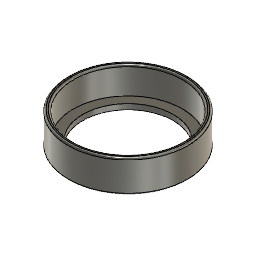
16) PLA Flexure Housing Ring 0.2mm Offset S2 (Autodesk Fusion 360 design; units mm, degrees)
Autodesk Fusion 360 part; units mm, degrees
sketch "Sketch1" plane through (0, 0, 0) normal (0, 0, 1) x (1, 0, 0)
  circle A0 centre (0, 0) radius 25
  circle A1 centre (0, 0) radius 30
  circle A2 centre (0, 0) radius 33
  dimension "d1" = 50
  dimension "d2" = 60
  dimension "d3" = 66
  constraint coincident A0.centre A1.centre
  constraint concentric A0 A1
  measures "d1" diameter of A0
  measures "d2" diameter of A1
  measures "d3" diameter of A2
extrude "Extrude1" add sketch "Sketch1" along normal blind 3 contours A1 | A2
sketch "Sketch2" plane through (0, 0, 3) normal (0, 0, 1) x (-1, 0, 0)
  circle A0 centre (0, 0) radius 25
  circle A1 centre (0, 0) radius 33
  circle A2 centre (0, 0) radius 30
  circle A3 centre (0, 0) radius 33
extrude "Extrude2" add sketch "Sketch2" along normal blind 15 contours A1 A3
fillet "Fillet1" radius 1 2 edges at (27.9698, -10.8485, 18) (30.7668, 11.9333, 18)
fillet "Fillet2" radius 1 1 edges at (-30.7668, -11.9333, 0)
move_face "OffsetFaces1" offset -0.2 1 faces at (-29.8509, 2.987, 7.6667)
named bodies: "Flexure Housing Ring 0.2mm Offset"
